Autodesk Inventor part; units mm, degrees
(part 2 of 2)
  spline S132 degree 2 poles (208.0885, -50.9333) (208.1176, -50.8091) (208.0662, -50.5391) (207.9855, -50.4037) knots 0 0 0 1 2 2 2
  line L126 (207.9855, -50.4037) -> (206.6894, -50.1008)
  line L127 (206.6894, -50.1008) -> (206.7613, -49.7931)
  line L128 (206.7613, -49.7931) -> (208.5881, -50.22)
  line L129 (208.5881, -50.22) -> (208.5162, -50.5277)
  line L130 (208.5162, -50.5277) -> (208.244, -50.4641)
  spline S133 degree 2 poles (208.244, -50.4641) (208.3547, -50.6668) (208.4185, -50.9459) (208.3908, -51.0643) knots 0 0 0 1 2 2 2
  spline S134 degree 2 poles (208.3908, -51.0643) (208.3797, -51.1117) (208.3647, -51.1581) (208.3519, -51.1863) knots 0 0 0 1 2 2 2
  line L131 (208.3519, -51.1863) -> (208.0323, -51.1116)
  spline S135 degree 2 poles (206.0621, -52.5251) (206.1072, -52.3422) (206.2836, -52.0497) (206.3644, -51.9591) knots 0 0 0 1 2 2 2
  line L132 (206.3644, -51.9591) -> (206.7087, -52.0439)
  line L133 (206.7087, -52.0439) -> (206.7048, -52.0597)
  spline S136 degree 2 poles (206.7048, -52.0597) (206.6636, -52.0912) (206.5627, -52.179) (206.4995, -52.2574) knots 0 0 0 1 2 2 2
  spline S137 degree 2 poles (206.4995, -52.2574) (206.4433, -52.3249) (206.3416, -52.5001) (206.3169, -52.6004) knots 0 0 0 1 2 2 2
  spline S138 degree 2 poles (206.3169, -52.6004) (206.2989, -52.6732) (206.2912, -52.8487) (206.309, -52.8948) knots 0 0 0 1 2 2 2
  spline S139 degree 2 poles (206.309, -52.8948) (206.3323, -52.961) (206.4043, -53.033) (206.4908, -53.0544) knots 0 0 0 1 2 2 2
  spline S140 degree 2 poles (206.4908, -53.0544) (206.599, -53.0811) (206.7402, -52.9907) (206.8149, -52.8484) knots 0 0 0 1 2 2 2
  spline S141 degree 2 poles (206.8149, -52.8484) (206.8433, -52.7928) (206.9292, -52.6137) (206.9707, -52.5384) knots 0 0 0 1 2 2 2
  spline S142 degree 2 poles (206.9707, -52.5384) (207.0831, -52.3449) (207.3814, -52.2181) (207.5604, -52.2623) knots 0 0 0 1 2 2 2
  spline S143 degree 2 poles (207.5604, -52.2623) (207.8083, -52.3234) (208.0254, -52.7713) (207.9498, -53.0782) knots 0 0 0 1 2 2 2
  spline S144 degree 2 poles (207.9498, -53.0782) (207.9124, -53.2296) (207.762, -53.518) (207.6793, -53.6082) knots 0 0 0 1 2 2 2
  line L134 (207.6793, -53.6082) -> (207.3508, -53.5272)
  line L135 (207.3508, -53.5272) -> (207.3546, -53.5115)
  spline S145 degree 2 poles (207.3546, -53.5115) (207.4782, -53.4168) (207.6572, -53.1563) (207.6935, -53.0087) knots 0 0 0 1 2 2 2
  spline S146 degree 2 poles (207.6935, -53.0087) (207.7309, -52.8573) (207.6544, -52.6172) (207.5266, -52.5857) knots 0 0 0 1 2 2 2
  spline S147 degree 2 poles (207.5266, -52.5857) (207.4105, -52.5571) (207.2678, -52.6534) (207.1985, -52.7823) knots 0 0 0 1 2 2 2
  spline S148 degree 2 poles (207.1985, -52.7823) (207.1643, -52.8448) (207.0872, -53.0053) (207.0427, -53.0924) knots 0 0 0 1 2 2 2
  spline S149 degree 2 poles (207.0427, -53.0924) (206.9421, -53.2804) (206.6576, -53.4273) (206.455, -53.3773) knots 0 0 0 1 2 2 2
  spline S150 degree 2 poles (206.455, -53.3773) (206.337, -53.3482) (206.1513, -53.2044) (206.0969, -53.095) knots 0 0 0 1 2 2 2
  spline S151 degree 2 poles (206.0969, -53.095) (206.04, -52.9787) (206.016, -52.712) (206.0621, -52.5251) knots 0 0 0 1 2 2 2
  spline S152 degree 2 poles (205.4148, -55.113) (205.4794, -54.864) (205.8364, -54.6573) (206.1443, -54.7371) knots 0 0 0 1 2 2 2
  line L136 (206.1443, -54.7371) -> (207.1504, -54.9979)
  line L137 (207.1504, -54.9979) -> (207.2038, -54.792)
  line L138 (207.2038, -54.792) -> (207.4567, -54.8576)
  line L139 (207.4567, -54.8576) -> (207.4034, -55.0635)
  line L140 (207.4034, -55.0635) -> (207.925, -55.1987)
  line L141 (207.925, -55.1987) -> (207.8457, -55.5047)
  line L142 (207.8457, -55.5047) -> (207.324, -55.3694)
  line L143 (207.324, -55.3694) -> (207.1781, -55.9323)
  line L144 (207.1781, -55.9323) -> (206.9251, -55.8667)
  line L145 (206.9251, -55.8667) -> (207.0711, -55.3038)
  line L146 (207.0711, -55.3038) -> (206.2062, -55.0796)
  spline S153 degree 2 poles (206.2062, -55.0796) (206.0689, -55.044) (205.9154, -55.0147) (205.842, -55.0312) knots 0 0 0 1 2 2 2
  spline S154 degree 2 poles (205.842, -55.0312) (205.778, -55.044) (205.6891, -55.1528) (205.6617, -55.2587) knots 0 0 0 1 2 2 2
  spline S155 degree 2 poles (205.6617, -55.2587) (205.6424, -55.3332) (205.6514, -55.4841) (205.657, -55.5191) knots 0 0 0 1 2 2 2
  line L147 (205.657, -55.5191) -> (205.6524, -55.5367)
  line L148 (205.6524, -55.5367) -> (205.3778, -55.4655)
  spline S156 degree 2 poles (205.3778, -55.4655) (205.3767, -55.3731) (205.395, -55.1895) (205.4148, -55.113) knots 0 0 0 1 2 2 2
  line L149 (204.6428, -58.1316) -> (204.7261, -57.8267)
  line L150 (204.7261, -57.8267) -> (204.9254, -57.8812)
  spline S157 degree 2 poles (204.9254, -57.8812) (204.8407, -57.7068) (204.7825, -57.42) (204.8252, -57.2637) knots 0 0 0 1 2 2 2
  spline S158 degree 2 poles (204.8252, -57.2637) (204.8572, -57.1464) (204.9925, -56.9587) (205.0974, -56.9054) knots 0 0 0 1 2 2 2
  spline S159 degree 2 poles (205.0974, -56.9054) (205.2027, -56.8502) (205.4822, -56.8341) (205.666, -56.8842) knots 0 0 0 1 2 2 2
  line L151 (205.666, -56.8842) -> (206.8405, -57.205)
  line L152 (206.8405, -57.205) -> (206.7573, -57.5099)
  line L153 (206.7573, -57.5099) -> (205.7254, -57.2281)
  spline S160 degree 2 poles (205.7254, -57.2281) (205.5808, -57.1886) (205.3853, -57.1583) (205.3048, -57.1762) knots 0 0 0 1 2 2 2
  spline S161 degree 2 poles (205.3048, -57.1762) (205.2243, -57.1942) (205.1251, -57.3036) (205.0926, -57.4228) knots 0 0 0 1 2 2 2
  spline S162 degree 2 poles (205.0926, -57.4228) (205.0622, -57.5342) (205.1203, -57.821) (205.1834, -57.9516) knots 0 0 0 1 2 2 2
  line L154 (205.1834, -57.9516) -> (206.5358, -58.3209)
  line L155 (206.5358, -58.3209) -> (206.4526, -58.6258)
  line L156 (206.4526, -58.6258) -> (204.6428, -58.1316)
  line L157 (205.6224, -61.5411) -> (204.0159, -60.3418)
  line L158 (204.0159, -60.3418) -> (204.0945, -60.0693)
  line L159 (204.0945, -60.0693) -> (206.0913, -59.9157)
  line L160 (206.0913, -59.9157) -> (205.9964, -60.2447)
  line L161 (205.9964, -60.2447) -> (204.4664, -60.3368)
  line L162 (204.4664, -60.3368) -> (205.7134, -61.2258)
  line L163 (205.7134, -61.2258) -> (205.6224, -61.5411)
  line L164 (204.5771, -65.0023) -> (202.9222, -63.9986)
  line L165 (202.9222, -63.9986) -> (203.0075, -63.7196)
  line L166 (203.0075, -63.7196) -> (204.5247, -63.7046)
  line L167 (204.5247, -63.7046) -> (203.2746, -62.8458)
  line L168 (203.2746, -62.8458) -> (203.3593, -62.5688)
  line L169 (203.3593, -62.5688) -> (205.2938, -62.658)
  line L170 (205.2938, -62.658) -> (205.1978, -62.9719)
  line L171 (205.1978, -62.9719) -> (203.7116, -62.865)
  line L172 (203.7116, -62.865) -> (204.971, -63.7139)
  line L173 (204.971, -63.7139) -> (204.8946, -63.9639)
  line L174 (204.8946, -63.9639) -> (203.3722, -63.9751)
  line L175 (203.3722, -63.9751) -> (204.6701, -64.6981)
  line L176 (204.6701, -64.6981) -> (204.5771, -65.0023)
  line L177 (201.9254, -67.1276) -> (202.0444, -66.7594)
  line L178 (202.0444, -66.7594) -> (202.8554, -66.5424)
  line L179 (202.8554, -66.5424) -> (202.3284, -65.8803)
  line L180 (202.3284, -65.8803) -> (202.4387, -65.5391)
  line L181 (202.4387, -65.5391) -> (203.1236, -66.4438)
  line L182 (203.1236, -66.4438) -> (204.2219, -66.1216)
  line L183 (204.2219, -66.1216) -> (204.103, -66.4899)
  line L184 (204.103, -66.4899) -> (203.2984, -66.7068)
  line L185 (203.2984, -66.7068) -> (203.8208, -67.3632)
  line L186 (203.8208, -67.3632) -> (203.7106, -67.7044)
  line L187 (203.7106, -67.7044) -> (203.0283, -66.8048)
  line L188 (203.0283, -66.8048) -> (201.9254, -67.1276)
  line L189 (202.8151, -70.3758) -> (200.7069, -68.5975)
  line L190 (200.7069, -68.5975) -> (200.8153, -68.277)
  line L191 (200.8153, -68.277) -> (201.4483, -68.8461)
  line L192 (201.4483, -68.8461) -> (203.3572, -68.7733)
  line L193 (203.3572, -68.7733) -> (203.2481, -69.0957)
  line L194 (203.2481, -69.0957) -> (201.7674, -69.1359)
  line L195 (201.7674, -69.1359) -> (202.9202, -70.0649)
  line L196 (202.9202, -70.0649) -> (202.8151, -70.3758)
  line L197 (200.1968, -72.176) -> (200.6556, -70.8771)
  line L198 (200.6556, -70.8771) -> (200.8772, -70.9553)
  line L199 (200.8772, -70.9553) -> (201.8534, -72.3401)
  line L200 (201.8534, -72.3401) -> (202.1665, -71.4537)
  line L201 (202.1665, -71.4537) -> (202.411, -71.5401)
  line L202 (202.411, -71.5401) -> (201.9718, -72.7837)
  line L203 (201.9718, -72.7837) -> (201.7597, -72.7088)
  line L204 (201.7597, -72.7088) -> (200.781, -71.3189)
  line L205 (200.781, -71.3189) -> (200.447, -72.2644)
  line L206 (200.447, -72.2644) -> (200.1968, -72.176)
  dimension "d24" = 7
  constraints: 2 end point, 2 point on circle, 2 point on line, 1 centre point, 1 other
  measures "d24" distance of L0.start L0.end
emboss "Emboss2" sketch "Sketch11" operation cut depth 2 direction (0, -1, 0) contours A1 L198 L199 L200 L201 L202 L203 L204 L205 L206 | S2 S3 S4 S5 L3 S6 S7 S8 L4 L5 S9 S10 S11 L6 A1 L8 S0 S1 | A1 S1 S2 | L189 L190 L191 A1 | A1 L191 L192 L193 L194 L195 L196 L189 | A1 L178 L179 L181 L182 L183 L184 L185 L186 L187 L188 | L12 L13 L14 S18 S19 S16 A1 S17 L10 | A1 S16 S17 | A1 L166 L167 L169 L170 L171 L172 L173 L174 L175 L176 L164 | S24 S25 S26 S27 S28 L16 L17 S29 S30 S31 S32 S33 L18 L19 S34 S35 A1 | A1 S35 S24 | S38 S39 S40 S41 S42 L22 L23 L24 A1 L21 S36 S37 | A1 S37 S38 | A1 L159 L160 L161 L162 L163 L157 | A1 L150 S157 S158 S159 L151 L152 L153 S160 S161 S162 L154 L155 L156 | S47 S48 S49 S50 L26 L27 S51 S52 S53 L28 L29 S54 S55 A1 | A1 S55 S47 | S157 S158 A1 | L38 L39 L40 L41 L42 S62 S63 L43 L31 S60 S61 L32 L33 L34 L35 L36 A1 | S156 S152 A1 | A1 S152 L136 L137 L138 L139 L140 L141 L142 L143 L144 L145 L146 S153 S154 S155 L147 L148 S156 | S67 L44 S68 S69 S70 S71 S72 L45 L46 L47 S73 A1 | A1 S73 S74 L48 L49 S64 S65 S66 S67 | S151 S135 A1 | A1 S135 L132 L133 S136 S137 S138 S139 S140 S141 S142 S143 S144 L134 L135 S145 S146 S147 S148 S149 S150 S151 | L55 L56 L57 S82 S83 L58 A1 L52 S79 S80 S81 L53 | A1 L128 L129 L130 S133 S134 L131 L125 S131 S132 L126 | L123 L119 L120 A1 | A1 L120 S122 S123 S124 S125 S126 L121 L122 L123 | L60 L61 L62 A1 | S122 S123 A1 | S88 L69 L70 L71 L72 L73 A1 | A1 L73 S84 S85 L67 L68 S86 S87 S88 | S114 S115 A1 | A1 S115 L113 L115 L116 L117 S116 S117 S114 | L83 L84 L85 L86 L87 L88 L89 L78 L79 L80 L81 A1 | L113 L114 L115 A1 | S106 S107 A1 | A1 S107 S108 S109 S106 | L91 L92 L93 A1 | A1 L106 S101 S102 S103 L107 L109 L110 L111 S104 S105 L112 | L97 S93 S94 S95 L98 L99 L100 L101 L102 S96 S97 S98 S99 S100 L103 L104 L94 S89 S90 S91 S92 L95 A1 | L63 L64 L65 L66 | L74 L75 L76 L77
sketch "Sketch12" plane through (0, 3, 0) normal (0, 1, 0) x (1, 0, 0)
  arc A0 (199.0691, -74.0748) -> (211.0224, -3) centre (-89.6277, 11.0207) ccw
  line L0 (199.0691, -74.0748) -> (208.4839, -75.8731)
  line L1 (208.4839, -75.8731) -> (219.4854, -6.1614)
  line L2 (219.4854, -6.1614) -> (219.1092, -3)
  line L3 (225, -3) -> (204.978, -3) projected
  line L4 (211.0224, -3) -> (219.1092, -3)
  point P0 (0, 0)
  constraints: 8 end point, 2 point on circle, 1 centre point, 1 horizontal, 1 point on line
extrude "Extrusion8" add sketch "Sketch12" against normal blind 2
sketch "Sketch13" plane through (0, 3, 0) normal (0, 1, 0) x (1, 0, 0)
  line L0 (112.5, -184.2834) -> (112.5, -171.3731) projected
  line L1 (225, -184.2834) -> (225, -3) projected
  line L2 (112.5, -184.2834) -> (225, -184.2834)
  line L3 (225, -184.2834) -> (225, -134.2834)
  line L4 (225, -134.2834) -> (112.5, -134.2834)
  line L5 (112.5, -134.2834) -> (112.5, -184.2834)
  point P0 (0, 0)
  dimension "d30" = 50
  constraints: 8 end point, 2 parallel, 1 horizontal, 1 perpendicular, 1 point on line
  measures "d30" distance of L3.end L2.end
extrude "Extrusion9" cut sketch "Sketch13" against normal blind 5
sketch "Sketch14" plane through (0, 3, 0) normal (0, 1, 0) x (1, 0, 0)
  point P0 (0, 0)
body "Solid1"
